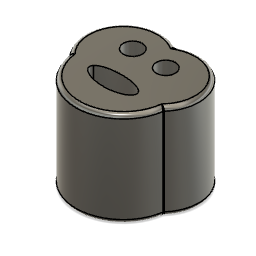
Shape 1 (Autodesk Fusion 360 design; units mm, degrees)
Autodesk Fusion 360 part; units mm, degrees
note: some values were not read from the file. Set by a fixed rule: which sketch regions a step uses.
sketch "Sketch1" plane through (0, 0, 0) normal (0, 1, 0) x (1, 0, 0)
  line L0 (-50, 50) -> (50, 50)
  line L1 (50, 50) -> (50, -50)
  line L2 (50, -50) -> (-50, -50)
  line L3 (-50, -50) -> (-50, 50)
  circle A0 centre (0, 0) radius 25
  circle A1 centre (-10, 10) radius 20
  circle A2 centre (10, 10) radius 20
  constraint horizontal L0
  constraint vertical L1
  constraint horizontal L2
  constraint vertical L3
  constraint coincident A0.centre origin
  constraint coincident A1 A2.centre
extrude "Extrude1" add sketch "Sketch1" along normal blind 50 contours A0 A1 A2 | A0 A1 A2 | A0 A1 A2 | A0 A1 A2 | A0 A1 A2 | A0 A1 A2 | A0 A1 A2
sketch "Sketch2" plane through (0, 0, 0) normal (0, 1, 0) x (1, 0, 0)
  circle A0 centre (-10, 15) radius 5
  circle A1 centre (7.4476, 15) radius 5
  spline S0 degree 5 poles (-12.7346, -3.0199) (-13.0446, -3.4092) (-13.4476, -4.2237) (-13.3778, -5.5224) (-11.9425, -7.262) (-8.2996, -9.0504) (-3.4504, -10.0964) (1.816, -10.1593) (6.666, -9.2134) (10.3191, -7.479) (12.1411, -5.3096) (11.7473, -3.1149) (9.1072, -1.2755) (4.6848, -0.0562) (-0.7175, 0.3899) (-6.1349, 0.0117) (-9.7049, -0.9119) (-11.5876, -1.8877) (-12.4246, -2.6305) (-12.7346, -3.0199) knots 0 0 0 0 0 0 0.066667 0.133333 0.2 0.266667 0.333333 0.4 0.466667 0.533333 0.6 0.666667 0.733333 0.8 0.866667 0.933333 1 1 1 1 1 1
  point P0 (0, -10)
  point P1 (11.0417, -3.0199)
  dimension "d3" = 10
  measures "d3" diameter of A1
extrude "Extrude2" cut sketch "Sketch2" along normal blind 50
fillet "Fillet1" radius 2 3 edges at (-25.5941, 50, -22.523) (25.5941, 50, -22.523) (0, 50, 25)
fillet "Fillet2" radius 1 6 edges at (24.7533, 24, 3.5033) (24.1816, 49.4314, 3.2332) (-24.7533, 24, 3.5033) (-24.1816, 49.4314, 3.2332) (0, 24, -27.3205) (0, 49.4713, -26.5712)
fillet "Fillet3" radius 2 6 edges at (25.6722, 0, -22.425) (0, 0, -27.4662) (-25.6722, 0, -22.425) (-24.7935, 0, 3.523) (0, 0, 25) (24.7935, 0, 3.523)
